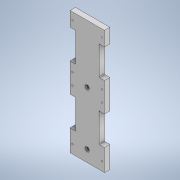
# Autodesk Inventor part: rail
Saved by Autodesk Inventor 2020 (Build 240168000, 168)
## iProperties
Created: 2019-12-19
Part Number: rail
Material: Générique
Document SubType Name: Modeling
Designer: damien
Density: 1 g/cm^3
Appearance: Par défaut
Author: damien
Autodesk Inventor part; units mm, degrees
ref_plane "YZ Plane" through (0, 0, 0) normal (1, 0, 0) x (0, 1, 0)
ref_plane "XZ Plane" through (0, 0, 0) normal (0, 1, 0) x (-1, 0, 0)
ref_plane "XY Plane" through (0, 0, 0) normal (0, 0, 1) x (1, 0, 0)
sketch "Esquisse1" plane through (0, 0, 0) normal (0, 0, 1) x (1, 0, 0)
  line L0 (0, 0) -> (-118.5, 0)
  line L1 (-118.5, 0) -> (-118.5, -425)
  line L2 (-118.5, -425) -> (0, -425)
  line L3 (0, -425) -> (0, 0)
  dimension "d0" = 425
  dimension "d3" = 118.5
  constraints: 8 end point, 3 perpendicular, 1 horizontal
  measures "d0" distance of L0.end L1.end
  measures "d3" distance of L0.start L0.end
extrude "Extrusion1" add sketch "Esquisse1" along normal blind 18.55
sketch "Esquisse2" plane through (0, 0, 18.55) normal (0, 0, 1) x (1, 0, 0)
  line L0 (-118.5, 0) -> (-118.5, -425) construction
  line L1 (-118.5, -50) -> (-99.95, -50)
  line L2 (-99.95, -50) -> (-99.95, -150)
  line L3 (-99.95, -150) -> (-118.5, -150)
  line L4 (-118.5, -150) -> (-118.5, -50)
  line L5 (-118.5, -250) -> (-99.95, -250)
  line L6 (-99.95, -250) -> (-99.95, -350)
  line L7 (-99.95, -350) -> (-118.5, -350)
  line L8 (-118.5, -350) -> (-118.5, -250)
  line L9 (0, 0) -> (-118.5, 0) projected
  line L10 (-118.5, -425) -> (0, -425) projected
  line L11 (-59.25, 0) -> (-59.25, -425) construction
  line L12 (0, 0) -> (0, -425) construction
  line L13 (0, -50) -> (-18.55, -50)
  line L14 (-18.55, -50) -> (-18.55, -150)
  line L15 (-18.55, -150) -> (0, -150)
  line L16 (0, -150) -> (0, -50)
  line L17 (0, -250) -> (-18.55, -250)
  line L18 (-18.55, -250) -> (-18.55, -350)
  line L19 (-18.55, -350) -> (0, -350)
  line L20 (0, -350) -> (0, -250)
  dimension "d27" = 18.55
  dimension "d28" = 100
  dimension "d29" = 100
  dimension "d30" = 100
  dimension "d31" = 50
  dimension "d32" = 75
  constraints: 36 end point, 8 symmetric about line, 4 parallel, 4 point on line, 2 horizontal, 2 midpoint, 2 perpendicular, 1 collinear
  measures "d27" distance of L2.end L3.end
  measures "d28" distance of L1.end L2.end
  measures "d29" distance of L5.end L6.end
  measures "d30" distance between parallel lines of L5 L3
  measures "d31" distance between parallel lines of L9 L1
  measures "d32" distance between parallel lines of L10 L7
extrude "Extrusion2" cut sketch "Esquisse2" against normal blind 18.55
sketch "Esquisse3" plane through (0, 0, 18.55) normal (0, 0, 1) x (1, 0, 0)
  line L0 (0, -425) -> (0, 0) projected
  line L1 (-118.5, -425) -> (0, -425) projected
  line L2 (-118.5, -350) -> (-118.5, -425) projected
  line L3 (-67.5329, -385) -> (-63.4915, -378)
  line L4 (-63.4915, -378) -> (-55.4085, -378)
  line L5 (-55.4085, -378) -> (-51.3671, -385)
  line L6 (-51.3671, -385) -> (-55.4085, -392)
  line L7 (-55.4085, -392) -> (-63.4915, -392)
  line L8 (-63.4915, -392) -> (-67.5329, -385)
  line L9 (-99.95, -250) -> (-99.95, -350) projected
  line L10 (-18.55, -350) -> (-18.55, -250) projected
  line L11 (-55.4085, -207) -> (-63.4915, -207)
  line L12 (-63.4915, -207) -> (-67.5329, -200)
  line L13 (-67.5329, -200) -> (-63.4915, -193)
  line L14 (-63.4915, -193) -> (-55.4085, -193)
  line L15 (-55.4085, -193) -> (-51.3671, -200)
  line L16 (-51.3671, -200) -> (-55.4085, -207)
  line L17 (-118.5, -150) -> (-118.5, -250) projected
  line L18 (-118.5, -200) -> (-59.45, -200) construction
  point P0 (-59.45, -385)
  dimension "d43" = 14
  dimension "d44" = 40.5
  dimension "d45" = 40.9
  dimension "d46" = 40
  constraints: 26 end point, 3 parallel, 1 horizontal, 1 midpoint, 1 vertical alignment, 26 other
  measures "d43" distance between parallel lines of L7 L4
  measures "d44" distance from line of L9 point (-59.45, -385)
  measures "d45" distance from line of point (-59.45, -385) L10
  measures "d46" distance from line of L1 point (-59.45, -385)
extrude "Extrusion3" cut sketch "Esquisse3" against normal blind 7
sketch "Esquisse4" plane through (0, 0, 18.55) normal (0, 0, 1) x (1, 0, 0)
  circle A0 centre (-101.0725, -51.1225) radius 1.5875
  circle A1 centre (-17.4275, -51.1225) radius 1.5875
  circle A2 centre (-101.0725, -148.8775) radius 1.5875
  circle A3 centre (-17.4275, -148.8775) radius 1.5875
  line L0 (-118.5, -50) -> (-99.95, -50) projected
  line L1 (-99.95, -50) -> (-101.0725, -51.1225) construction
  line L2 (-99.95, -150) -> (-99.95, -50) projected
  line L3 (-101.0725, -148.8775) -> (-99.95, -150) construction
  line L4 (-99.95, -150) -> (-118.5, -150) projected
  line L5 (-18.55, -50) -> (0, -50) projected
  line L6 (-18.55, -50) -> (-17.4275, -51.1225) construction
  line L7 (-18.55, -150) -> (-18.55, -50) projected
  line L8 (-18.55, -150) -> (-17.4275, -148.8775) construction
  line L9 (0, -150) -> (-18.55, -150) projected
  line L10 (-118.5, -150) -> (-118.5, -250) projected
  line L11 (-118.5, -200) -> (0, -200) construction
  line L12 (0, -250) -> (0, -150) projected
  circle A4 centre (-101.0725, -348.8775) radius 1.5875
  circle A5 centre (-17.4275, -348.8775) radius 1.5875
  circle A6 centre (-101.0725, -251.1225) radius 1.5875
  circle A7 centre (-17.4275, -251.1225) radius 1.5875
  line L13 (-99.95, -350) -> (-101.0725, -348.8775) construction
  line L14 (-101.0725, -251.1225) -> (-99.95, -250) construction
  line L15 (-18.55, -350) -> (-17.4275, -348.8775) construction
  line L16 (-18.55, -250) -> (-17.4275, -251.1225) construction
  point P0 (0, 0)
  point P1 (-99.95, -350)
  point P2 (-99.95, -250)
  point P3 (-18.55, -350)
  point P4 (-18.55, -250)
  dimension "d34" = 3.175
  dimension "d51" = 45
  dimension "d52" = 45
  dimension "d53" = 45
  dimension "d54" = 45
  constraints: 18 end point, 8 symmetric about line, 4 horizontal, 2 midpoint, 24 other
  measures "d51" angle of L4 L3
  measures "d52" angle of L6 L5
  measures "d53" angle of L9 L8
  measures "d54" angle of L2 L1
extrude "Extrusion4" cut sketch "Esquisse4" against normal blind 18.55
sketch "Esquisse5" plane through (0, 0, 18.55) normal (0, 0, 1) x (1, 0, 0)
  circle A0 centre (-110.3475, -25) radius 2.25
  circle A1 centre (-110.3475, -180) radius 2.25
  circle A2 centre (-110.3475, -395) radius 2.25
  line L0 (-118.5, -50) -> (-102.1951, -50) projected
  line L1 (-110.3475, -50) -> (-110.3475, -425) construction
  line L2 (-118.5, -425) -> (0, -425) projected
  line L3 (-110.3475, -50) -> (-110.3475, 0) construction
  line L4 (0, 0) -> (-118.5, 0) projected
  line L5 (-99.95, -350) -> (-118.5, -350) projected
  line L6 (-102.1951, -150) -> (-118.5, -150) projected
  line L7 (-59.25, 0) -> (-59.25, -425) construction
  circle A3 centre (-8.1525, -25) radius 2.25
  circle A4 centre (-8.1525, -180) radius 2.25
  circle A5 centre (-8.1525, -395) radius 2.25
  line L8 (0, -50) -> (-16.3049, -50)
  line L9 (-8.1525, -50) -> (-8.1525, -425) construction
  line L10 (-8.1525, -50) -> (-8.1525, 0) construction
  line L11 (-16.9625, -350.1) -> (0, -350)
  line L12 (-16.3049, -150) -> (0, -150)
  circle A6 centre (-110.3475, -220) radius 2.25
  line L13 (-118.5, -250) -> (-102.1951, -250) projected
  circle A7 centre (-8.1525, -220) radius 2.25
  point P0 (-101.5375, -350.1)
  dimension "d37" = 4.5
  dimension "d38" = 30
  dimension "d39" = 45
  dimension "d40" = 30
  dimension "d56" = 30
  constraints: 16 end point, 13 symmetric about line, 8 centre point, 7 point on line, 6 midpoint, 3 equal radius, 2 vertical, 5 other
  measures "d37" diameter of A0
  measures "d38" distance from line of L2 A2.centre
  measures "d40" distance from line of A1.centre L6
  measures "d56" distance from line of A6.centre L13
extrude "Extrusion5" cut sketch "Esquisse5" against normal blind 120
sketch "Esquisse6" plane through (0, 0, 11.55) normal (0, 0, 1) x (1, 0, 0)
  circle A0 centre (-59.45, -385) radius 5.25
  line L0 (-63.4915, -392) -> (-67.5329, -385) projected
  line L1 (-63.4915, -378) -> (-55.4085, -378) projected
  line L2 (-63.4915, -392) -> (-55.4085, -378) construction
  line L3 (-63.4915, -378) -> (-55.4085, -392) construction
  circle A1 centre (-59.45, -200) radius 5.25
  line L4 (-63.4915, -193) -> (-55.4085, -207) construction
  point P0 (0, 0)
  dimension "d47" = 10.5
  constraints: 6 end point, 3 midpoint, 2 centre point, 2 coincident, 1 equal radius, 1 vertical alignment
  measures "d47" diameter of A0
extrude "Extrusion6" cut sketch "Esquisse6" against normal blind 18
sketch "Esquisse7" plane through (0, 0, 0) normal (0, 0, -1) x (-1, 0, 0)
  circle A0 centre (59.45, -200) radius 5.25 construction
  circle A1 centre (59.45, -200) radius 30
  circle A2 centre (59.45, -385) radius 5.25 construction
  circle A3 centre (59.45, -385) radius 30
  point P0 (0, 0)
  dimension "d57" = 60
  constraints: 2 centre point, 2 coincident, 1 equal radius
  measures "d57" diameter of A1
extrude "Extrusion7" cut sketch "Esquisse7" against normal blind 2.5
